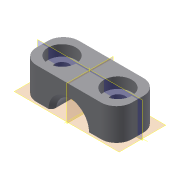
# Autodesk Inventor part: Cycl_fijadorVarillaLisah
Saved by Autodesk Inventor 2015 SP2 (Build 190223200, 223)
## iProperties
Created: 2015-04-21
Material: Genérico
Document SubType Name: Modeling
Designer: E.Beroiz
Density: 1 g/cm^3
Appearance: Valor por defecto
Description: Cycl_fijadorVarillaLisah
Author: E.Beroiz
Autodesk Inventor part; units mm, degrees
sketch "Boceto1" plane through (0, 0, 0) normal (0, 0, 1) x (1, 0, 0)
  line L0 (-12.375, 5.5) -> (12.375, 5.5)
  line L1 (12.375, 5.5) -> (12.375, -5.5)
  line L2 (12.375, -5.5) -> (-12.375, -5.5)
  line L3 (-12.375, -5.5) -> (-12.375, 5.5)
  point P0 (0, 0)
  point P1 (12.375, 0)
  point P2 (0, 5.5)
  dimension "d0" = 24.75
  dimension "d1" = 11
  constraints: 8 end point, 2 midpoint, 2 parallel, 1 horizontal, 1 horizontal alignment, 1 perpendicular, 1 vertical alignment
  measures "d0" distance of L1.end L2.end
  measures "d1" distance of L0.end L1.end
extrude "Extrusión1" add sketch "Boceto1" along normal blind 8.25
sketch "Boceto2" plane through (0, 0, 8.25) normal (0, 0, 1) x (1, 0, 0)
  circle A0 centre (-7.25, 0) radius 3.6
  circle A1 centre (7.25, 0) radius 3.6
  point P0 (0, 0)
  dimension "d4" = 7.2
  dimension "d5" = 7.2
  dimension "d6" = 7.3
  dimension "d7" = 7.25
  constraints: 2 centre point, 2 horizontal alignment
  measures "d4" diameter of A0
  measures "d5" diameter of A1
  measures "d7" distance of point (0, 0) A1.centre
extrude "Extrusión2" cut sketch "Boceto2" against normal blind 2.79
hole "Agujero1" at (-7.25, 0, 5.46) direction (0, 0, -1) diameter 3.78 end through all
hole "Agujero2" at (7.25, 0, 5.46) direction (0, 0, -1) diameter 3.78 end through all
fillet "Empalme1" radius 4 4 edges at (12.375, -5.5, 4.125) (12.375, 5.5, 4.125) (-12.375, -5.5, 4.125) (-12.375, 5.5, 4.125)
sketch "Boceto3" plane through (-8.375, -5.5, 0) normal (0, -1, 0) x (1, 0, 0)
  line L0 (16.75, 0) -> (0, 0) projected
  arc A0 (12.625, 0) -> (4.125, 0) centre (8.375, 0) ccw
  line L1 (4.125, 0) -> (12.625, 0)
  point P0 (8.375, 4.25)
  dimension "d34" = 4.25
  constraints: 3 point on circle, 2 coincident, 2 end point, 2 midpoint, 2 point on line, 1 centre point, 1 collinear
  measures "d34" radius of A0
extrude "Extrusión3" cut sketch "Boceto3" against normal through all
chamfer "Chaflán1" distance 1 angle 45 2 edges at (0, -5.5, 4.25) (0, 5.5, 4.25) measured on face at (-4.2362, -1.8333, 0.342)
fillet "Empalme2" radius 0.5 2 edges at (-4.25, 0, 0) (4.25, 0, 0)
